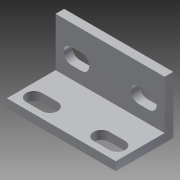
# Autodesk Inventor part: L bracket double
Saved by Autodesk Inventor 2014 SP1 (Build 180222100, 222)
## iProperties
Created: 2016-04-18
Part Number: L bracket double
Material: Generic
Document SubType Name: Modeling
Designer: Ben
Density: 1 g/cm^3
Appearance: Default
Author: Ben
Autodesk Inventor part; units mm, degrees
ref_plane "YZ Plane" through (0, 0, 0) normal (1, 0, 0) x (0, 1, 0)
ref_plane "XZ Plane" through (0, 0, 0) normal (0, 1, 0) x (-1, 0, 0)
ref_plane "XY Plane" through (0, 0, 0) normal (0, 0, 1) x (1, 0, 0)
sketch "Sketch1" plane through (0, 0, 0) normal (0, 0, 1) x (1, 0, 0)
  line L0 (-19, 10) -> (19, 10)
  line L1 (19, 10) -> (19, -10)
  line L2 (19, -10) -> (-19, -10)
  line L3 (-19, -10) -> (-19, 10)
  line L4 (-19, 0) -> (19, 0) construction
  line L5 (-13.5, 0) -> (-10, 0) construction
  line L6 (-13.5, -2.75) -> (-10, -2.75)
  line L7 (-10, 2.75) -> (-13.5, 2.75)
  arc A0 (-13.5, 2.75) -> (-13.5, -2.75) centre (-13.5, 0) ccw
  arc A1 (-10, -2.75) -> (-10, 2.75) centre (-10, 0) ccw
  line L8 (0, 10) -> (0, -10) construction
  line L9 (13.5, 0) -> (10, 0) construction
  line L10 (13.5, -2.75) -> (10, -2.75)
  line L11 (10, 2.75) -> (13.5, 2.75)
  arc A2 (13.5, -2.75) -> (13.5, 2.75) centre (13.5, 0) ccw
  arc A3 (10, 2.75) -> (10, -2.75) centre (10, 0) ccw
  point P0 (0, 0)
  point P1 (-11.75, 0)
  point P2 (11.75, 0)
  dimension "d0" = 20
  dimension "d1" = 38
  dimension "d2" = 5.5
  dimension "d3" = 3.5
  dimension "d4" = 10
  dimension "d15" = 23.5
  constraints: 28 end point, 8 point on circle, 7 midpoint, 7 symmetric about line, 4 centre point, 4 tangent, 3 parallel, 2 point on line, 1 horizontal, 1 perpendicular, 2 other
  measures "d0" distance of L2.end L0.start
  measures "d1" distance of L0.start L0.end
  measures "d2" diameter of A1
  measures "d3" distance of L5.end L5.start
  measures "d4" distance between parallel lines of L0 L4
  measures "d15" distance of point (11.75, 0) point (-11.75, 0)
extrude "Extrusion1" add sketch "Sketch1" along normal blind 3
sketch "Sketch2" plane through (0, 0, 3) normal (0, 0, 1) x (1, 0, 0)
  line L0 (19, -10) -> (19, 10) projected
  line L1 (-19, -10) -> (19, -10)
  line L2 (19, -10) -> (19, -7)
  line L3 (19, -7) -> (-19, -7)
  line L4 (-19, -7) -> (-19, -10)
  point P0 (0, 0)
  dimension "d7" = 3
  constraints: 8 end point, 2 parallel, 1 horizontal, 1 perpendicular, 1 point on line
  measures "d7" distance of L1.end L2.end
extrude "Extrusion2" add sketch "Sketch2" along normal blind 17
sketch "Sketch3" plane through (-19, -7, 3) normal (0, 1, 0) x (1, 0, 0)
  line L0 (0, 0) -> (0, -17) projected
  line L1 (38, -17) -> (0, -17) projected
  line L2 (38, 0) -> (38, -17) projected
  line L3 (0, -12) -> (38, -12) construction
  line L4 (4.5, -12) -> (10, -12) construction
  line L5 (4.5, -14.75) -> (10, -14.75)
  line L6 (10, -9.25) -> (4.5, -9.25)
  arc A0 (4.5, -9.25) -> (4.5, -14.75) centre (4.5, -12) ccw
  arc A1 (10, -14.75) -> (10, -9.25) centre (10, -12) ccw
  line L7 (0, 0) -> (38, 0) projected
  line L8 (19, 0) -> (19, -17) construction
  line L9 (33.5, -12) -> (28, -12) construction
  line L10 (33.5, -14.75) -> (28, -14.75)
  line L11 (28, -9.25) -> (33.5, -9.25)
  arc A2 (33.5, -14.75) -> (33.5, -9.25) centre (33.5, -12) ccw
  arc A3 (28, -9.25) -> (28, -14.75) centre (28, -12) ccw
  point P0 (19, 3)
  point P1 (7.25, -12)
  point P2 (19, -12)
  point P3 (30.75, -12)
  dimension "d10" = 5.5
  dimension "d11" = 5.5
  dimension "d12" = 5
  dimension "d16" = 23.5
  constraints: 20 end point, 8 point on circle, 7 symmetric about line, 4 centre point, 4 midpoint, 4 point on line, 4 tangent, 1 parallel, 1 perpendicular, 2 other
  measures "d10" diameter of A1
  measures "d11" distance of L4.end L4.start
  measures "d12" distance between parallel lines of L1 L3
  measures "d16" distance of point (30.75, -12) point (7.25, -12)
extrude "Extrusion3" cut sketch "Sketch3" against normal up to surface (3 mm away) contours A0 L6 A1 L5 | L10 A3 L11 A2
body "Solid1"
